Autodesk Inventor part; units mm, degrees
(part 2 of 2)
sketch "Sketch2" plane through (0, 0, 0) normal (0, 1, 0) x (-1, 0, 0)
  line L0 (-1278471.3795, 0) -> (-3471.3795, 0) construction
  line L1 (-3471.3795, 0) -> (-3471.3795, -1090759.1919) construction
  line L2 (-3471.3795, -1090759.1919) -> (-1278471.3795, -1090759.1919) construction
  line L3 (-1278471.3795, -1090759.1919) -> (-1278471.3795, 0) construction
  line L4 (-4892.4841, -1049180.2136) -> (-1275042.0064, -796354.188)
  line L5 (-1275042.0064, -796354.188) -> (-1275042.0064, -777036.7977)
  line L6 (-1275042.0064, -777036.7977) -> (-1106336.8035, -815242.3029)
  line L7 (-1106336.8035, -815242.3029) -> (-1036931.059, -538201.2489)
  line L8 (-1036931.059, -538201.2489) -> (-968295.3087, -548177.3753)
  line L9 (-968295.3087, -548177.3753) -> (-938708.0677, -344617.1564)
  line L10 (-938708.0677, -344617.1564) -> (-905497.1449, -349444.3254)
  line L11 (-905497.1449, -349444.3254) -> (-914495.6977, -411354.3689)
  line L12 (-914495.6977, -411354.3689) -> (-827707.617, -428629.7252)
  line L13 (-827707.617, -428629.7252) -> (-797910.3728, -248065.5725)
  line L14 (-797910.3728, -248065.5725) -> (-702190.2619, -257789.5373)
  line L15 (-702190.2619, -257789.5373) -> (-689475.0202, -207035.1798)
  line L16 (-689475.0202, -207035.1798) -> (-512498.2646, -225013.8023)
  line L17 (-512498.2646, -225013.8023) -> (-468044.8652, -6617.0395)
  line L18 (-468044.8652, -6617.0395) -> (-459749.1046, -5862.8794)
  line L19 (-459749.1046, -5862.8794) -> (-479378.6175, -102301.4451)
  line L20 (-479378.6175, -102301.4451) -> (-196609.4051, -146484.5316)
  line L21 (-196609.4051, -146484.5316) -> (-191430.6505, -129630.041)
  line L22 (-191430.6505, -129630.041) -> (-174387.8397, -129630.041)
  line L23 (-174387.8397, -129630.041) -> (-173027.5023, -135284.6402)
  line L24 (-173027.5023, -135284.6402) -> (-189076.6711, -135284.6402)
  line L25 (-189076.6711, -135284.6402) -> (-199471.9628, -237613.1144)
  line L26 (-199471.9628, -237613.1144) -> (-150218.1122, -247417.2005)
  line L27 (-150218.1122, -247417.2005) -> (-137887.1302, -185468.7093)
  line L28 (-137887.1302, -185468.7093) -> (-128507.5049, -181561.8305)
  line L29 (-128507.5049, -181561.8305) -> (-123030.6256, -190850.621)
  line L30 (-123030.6256, -190850.621) -> (-124605.017, -198760.0617)
  line L31 (-124605.017, -198760.0617) -> (-133197.3176, -203826.275)
  line L32 (-133197.3176, -203826.275) -> (-139314.6967, -242977.1496)
  line L33 (-139314.6967, -242977.1496) -> (-130727.7376, -250174.8579)
  line L34 (-130727.7376, -250174.8579) -> (-154761.9111, -433319.9435)
  line L35 (-154761.9111, -433319.9435) -> (-118222.3298, -440593.2267)
  line L36 (-118222.3298, -440593.2267) -> (-118222.3298, -242977.1496)
  line L37 (-118222.3298, -242977.1496) -> (-86013.3086, -4882.7115)
  line L38 (-86013.3086, -4882.7115) -> (-87721.181, -4651.6733)
  line L39 (-87721.181, -4651.6733) -> (-121339.7207, -253165.5071)
  line L40 (-121339.7207, -253165.5071) -> (-93669.1101, -598130.6676)
  line L41 (-93669.1101, -598130.6676) -> (-106431.2873, -922767.2008)
  line L42 (-106431.2873, -922767.2008) -> (-118222.3298, -1009928.5468)
  line L43 (-118222.3298, -1009928.5468) -> (-6212.1968, -1032727.5623)
  line L44 (-6212.1968, -1032727.5623) -> (-4892.4841, -1049180.2136)
  line L45 (-671212.042, -859953.6514) -> (-647404.5421, -683964.6551)
  line L46 (-647404.5421, -683964.6551) -> (-630588.1488, -686239.5489)
  line L47 (-630588.1488, -686239.5489) -> (-620605.1309, -612443.4214)
  line L48 (-620605.1309, -612443.4214) -> (-549648.3449, -619651.7424)
  line L49 (-549648.3449, -619651.7424) -> (-584542.4472, -877594.7467)
  line L50 (-584542.4472, -877594.7467) -> (-671212.042, -859953.6514)
  line L51 (-695681.5604, -854973.0223) -> (-659879.2223, -675108.9338)
  line L52 (-659879.2223, -675108.9338) -> (-683924.6707, -670322.635)
  line L53 (-683924.6707, -670322.635) -> (-674158.6609, -598130.6676)
  line L54 (-674158.6609, -598130.6676) -> (-742311.0203, -588911.1294)
  line L55 (-742311.0203, -588911.1294) -> (-775612.7223, -756212.5012)
  line L56 (-775612.7223, -756212.5012) -> (-749486.9391, -764239.9774)
  line L57 (-749486.9391, -764239.9774) -> (-755836.6185, -796139.5503)
  line L58 (-755836.6185, -796139.5503) -> (-784010.1212, -798399.4249)
  line L59 (-784010.1212, -798399.4249) -> (-791393.3669, -835491.437)
  line L60 (-695599.2412, -854559.4661) -> (-791393.3669, -835491.437)
  line L61 (-576818.3354, -887092.9743) -> (-575116.2202, -878541.8735)
  line L62 (-575116.2202, -878541.8735) -> (-537320.6136, -886065.1713)
  line L63 (-537320.6136, -886065.1713) -> (-542632.0179, -912748.649)
  line L64 (-542632.0179, -912748.649) -> (-516660.5915, -917918.3179)
  line L65 (-516660.5915, -917918.3179) -> (-508628.1772, -891776.4631)
  line L66 (-508628.1772, -891776.4631) -> (-573766.6415, -871761.849)
  line L67 (-573766.6415, -871761.849) -> (-555515.4249, -780071.2327)
  line L68 (-323937.3031, -821661.8474) -> (-342217.4744, -913497.9264)
  line L69 (-342217.4744, -913497.9264) -> (-227671.5266, -928993.5125)
  line L70 (-227671.5266, -928993.5125) -> (-214310.4379, -843483.3134)
  line L71 (-214310.4379, -843483.3134) -> (-323937.3031, -821661.8474)
  point P0 (0, 0)
  point P1 (0, 0)
  dimension "d5" = 1275000
  constraints: 136 end point, 27 perpendicular, 19 parallel, 14 point on line, 1 vertical, 2 other
  measures "d5" distance between parallel lines of L3 L1
extrude "Extrusion1" add sketch "Sketch1" along normal blind 122000 contours L4 L5 L6 L7 | L8 L9 L10 L11 L12 L13 L14 L15 L16 L17 L18 L19 L20 L21 L22 L23 L24 L25 L26 L27 L28 L29 L30 L31 L32 L33 L34 L35 L36 L37 L38 L39 L40 L41 L42 L43 L44 L45 L46 L47 L48 L49 L50 L51 L52 L53 | L54 L55 L56 L57 | L58 L59 L60 L61 | L62 L63 L64 L65 | L66 L67 L68 L69 L70 L71 | L72 L73 L74 L75 | L79 L78 L77 L76 | L80 L81 L82 L83 L84 L85 L86 L87 L88 L89 L90 L91 L92 L93 L94 L95 L96 L97 L98 L99 L100 L101 L102 L103 | L138 L137 L136 L135 | L139 L140 L141 L142 | L170 L169 L168 L167 L166 L165 L164 L163 L162 L161 L160 L159 L158 L157 L156 L155 L154 L153 L152 L151 L150 L149 L148 L147 L146 L145 L144 L143 | L179 L178 L177 L176 L175 L174 L173 L172 L171 | L180 L181 L182 L183 L184 L185 L186 L193 L192 L191 L190 L189 L188 L187 | L208 L209 L210 L211 L212 L213 L214 L215 L216 L217 L218 L219 L220 | L221 L222 L223 L224 L225 L226 L227 L228 L229 L230 L231 L232 L233 L234 L235 | L236 L237 L238 L239 L240 | L241 L242 L243 L244 L245 L246 L247 L248 L249 L250 L251 L252 L253 L254 L255 L256 L257 L258 L259 L260 L262 L261 | L268 L267 L266 L265 L264 L263 | L303 L302 L301 L300 L299 L298 L297 L296 L295 L294 L293 L292 L291 L290 L289 L288 L287 L286 L285 L284 L283 L282 L281 L280 L279 L278 L277 L276 L275 L274 L273 L272 L271 L270 L269 | L304 L305 L306 L307 | L311 L310 L309 L308 | L312 L313 L314 L315 | L316 L317 L318 L319 | L323 L322 L321 L320 | L327 L326 L325 L324 | L328 L329 L330 L331 L332 L333 L334 L335 L336 L337 L338 | L345 L344 L343 L346 L342 L341 L340 L339 | L354 L353 L352 L351 L350 L349 L348 L347 | L365 L364 L363 L362 | L366 L367 L368 L369 | L377 L376 L375 L374 L373 L372 L371 L370 | L404 L403 L402 L401 | L405 L406 L407 L408 | L416 L415 L414 L413 L412 L411 L410 L409 | L423 L422 L421 L420 L419 L418 L417 | L424 L425 L426 L427 | L435 L434 L433 L432 L431 L430 L429 L428 | L441 L439 L438 L437 L436 | L442 L443 L444 L445 L446 L447 | L451 L450 L449 L448 | L452 L453 L454 L455 L456 L457 L458 L459 L460 L461 | L462 L463 L464 L465 | L466 L467 L468 L469 | L473 L472 L471 L470 | L476 L477 L475 L474 | L478 L479 L480 L481 L482 | L483 L484 L485 L486 L487 L488 L489 L490 | L491 L492 L493 L494 L495 L496 L497 L498 | L504 L503 L502 L501 | L508 L507 L509 L506 | L513 L512 L511 L510 | L517 L516 L515 L514 | L530 L529 L528 L527 L526 L525 | L538 L537 L536 L535 L534 L533 L532 L531 | L542 L541 L540 L539 | L551 L550 L549 L548 L547 L546 L545 L544 L543 | L552 L555 L554 L553 | L556 L557 L558 L559 | L563 L562 L561 L560 | L564 L565 L566 L567 | L568 L569 L570 L571 | L575 L574 L573 L572 | L579 L578 L577 L576 | L580 L581 L582 L583 | L589 L588 L587 L586 L585 L584 | L595 L594 L593 L592 L591 L590 | L596 L597 L598 L599 L600 | L601 L602 L603 L604 | L608 L607 L606 L605 | L610 L611 L612 L613 | L614 L615 L616 L617 | L621 L620 L619 L618
body "Solid1"
